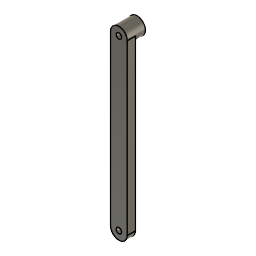
part - head link 1 (Autodesk Fusion 360 design; units mm, degrees)
Autodesk Fusion 360 part; units mm, degrees
sketch "Sketch1" plane through (0, 0, 0) normal (0, 1, 0) x (1, 0, 0)
  circle A0 centre (0, 0) radius 5
  circle A1 centre (0, 0) radius 1.6
  line L0 (-5, 0) -> (5, 0)
  line L1 (5, 0) -> (5, -100.7)
  line L2 (5, -100.7) -> (-5, -100.7)
  line L3 (-5, -100.7) -> (-5, 0)
  circle A2 centre (0, -100.7) radius 5
  circle A3 centre (0, -100.7) radius 1.6
  dimension "d1" = 10
  dimension "d2" = 3.2
  dimension "d3" = 100.7
  dimension "d4" = 3.2
  constraint coincident A0.centre A1.centre
  constraint perpendicular L0 L1
  constraint parallel L0 L2
  constraint parallel L1 L3
  constraint coincident A0 L0.end
  constraint horizontal L0
  constraint coincident A0 L0.start
  constraint midpoint L2 A2.centre
  constraint coincident L1.end A2
  constraint concentric A2 A3
  measures "d1" diameter of A0
  measures "d2" diameter of A1
  measures "d3" distance of L0.start L2.end
  measures "d4" diameter of A3
extrude "Extrude1" add sketch "Sketch1" along normal blind 5.9 contours L2 A2 A3 | L2 A2 A3
extrude "Extrude2" add sketch "Sketch1" against normal blind 5 contours A0 A1 L0 | A0 L1 L3 A2 | A0 A1 L0 | L2 A2 A3 | L2 A2 A3
equation "d3 = 106 mm - 20.3 mm + 15 mm"
